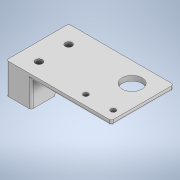
# Autodesk Inventor part: SwerveDriveBracket_B
Saved by Autodesk Inventor 2022.3 (Build 263350000, 350)
## iProperties
Created: 2022-06-17
Part Number: SwerveDriveBracket_B
Material: Generic
Document SubType Name: Modeling
Designer: Robert Nies
Density: 1 g/cm^3
Appearance: Default
Author: Robert Nies
Autodesk Inventor part; units mm, degrees
ref_plane "YZ Plane" through (0, 0, 0) normal (1, 0, 0) x (0, 1, 0)
ref_plane "XZ Plane" through (0, 0, 0) normal (0, 1, 0) x (-1, 0, 0)
ref_plane "XY Plane" through (0, 0, 0) normal (0, 0, 1) x (1, 0, 0)
sketch "Sketch1" plane through (0, 0, 0) normal (0, 1, 0) x (-1, 0, 0)
  line L0 (0, 0) -> (67.31, 0)
  line L1 (67.31, 0) -> (67.31, -40.005)
  line L2 (67.31, -40.005) -> (0, -40.005)
  line L3 (0, -40.005) -> (0, 0)
  dimension "d0" = 40.005
  dimension "d1" = 67.31
  constraints: 8 end point, 2 parallel, 1 horizontal, 1 perpendicular
  measures "d0" distance of L0.end L1.end
  measures "d1" distance of L1.end L2.end
extrude "Extrusion1" add sketch "Sketch1" along normal blind 3.175
sketch "Sketch2" plane through (0, 3.175, 0) normal (0, 1, 0) x (1, 0, 0)
  circle A0 centre (-13.97, 27.305) radius 6.35
  line L0 (0, 0) -> (0, 40.005) projected
  line L1 (-67.31, 0) -> (0, 0) projected
  line L2 (0, 40.005) -> (-67.31, 40.005) projected
  circle A1 centre (-5.08, 6.35) radius 1.5875
  circle A2 centre (-22.68, 6.35) radius 1.5875
  dimension "d4" = 13.97
  dimension "d28" = 12.7
  dimension "d29" = 12.7
  dimension "d30" = 3.175
  dimension "d31" = 3.175
  dimension "d32" = 5.08
  dimension "d33" = 17.6
  dimension "d34" = 6.35
  dimension "d35" = 6.35
  constraints: 3 centre point
  measures "d4" distance from line of L0 A0.centre
  measures "d28" distance from line of L2 A0.centre
  measures "d29" diameter of A0
  measures "d30" diameter of A1
  measures "d31" diameter of A2
  measures "d32" distance from line of L0 A1.centre
  measures "d33" distance of A1.centre A2.centre
  measures "d34" distance from line of L1 A1.centre
  measures "d35" distance from line of L1 A2.centre
extrude "Extrusion2" cut sketch "Sketch2" against normal blind 6.35
sketch "Sketch3" plane through (0, 0, 0) normal (0, -1, 0) x (1, 0, 0)
  line L0 (0, -40.005) -> (-67.31, -40.005) projected
  line L1 (-67.31, 0) -> (0, 0) projected
  line L2 (-67.31, -40.005) -> (-51.435, -40.005)
  line L3 (-51.435, -40.005) -> (-51.435, 0)
  line L4 (-51.435, 0) -> (-67.31, 0)
  line L5 (-67.31, 0) -> (-67.31, -40.005)
  point P0 (-67.31, 0)
  dimension "d8" = 15.875
  constraints: 8 end point, 2 parallel, 1 horizontal, 1 perpendicular, 1 point on line
  measures "d8" distance of L4.end L3.end
extrude "Extrusion3" add sketch "Sketch3" along normal blind 16.51
sketch "Sketch4" plane through (-67.31, 3.175, -40.005) normal (-1, 0, 0) x (0, 0, 1)
  line L0 (40.005, -19.685) -> (0, -19.685) projected
  circle A0 centre (20.0025, -19.685) radius 6.35
  point P0 (40.005, -3.175)
  point P1 (13.6525, -19.685)
  point P2 (26.3525, -19.685)
  dimension "d11" = 12.7
  constraints: 1 centre point, 1 midpoint
  measures "d11" diameter of A0
extrude "Extrusion4" cut sketch "Sketch4" against normal blind 6.35 contours L0 A0 picked at (22.0577, -19.1784)
sketch "Sketch5" plane through (-60.96, 3.175, -40.005) normal (-1, 0, 0) x (0, 0, 1)
  line L0 (26.3525, -19.685) -> (13.6525, -19.685) projected
  line L1 (20.0025, -19.685) -> (20.0025, -3.683)
  circle A0 centre (20.0025, -3.683) radius 3.175
  arc A1 (26.3525, -19.685) -> (13.6525, -19.685) centre (20.0025, -19.685) ccw projected
  line L2 (24.765, -15.4849) -> (15.24, -15.4849)
  line L3 (24.765, -15.4849) -> (23.1501, -3.267)
  line L4 (15.24, -15.4849) -> (16.8549, -3.267)
  point P0 (40.005, -3.175)
  dimension "d14" = 16.002
  dimension "d15" = 6.35
  dimension "d16" = 9.525
  constraints: 8 end point, 4 point on circle, 2 tangent, 1 centre point, 1 coincident, 1 horizontal, 1 midpoint, 1 vertical
  measures "d14" distance of L1.start L1.end
  measures "d15" diameter of A0
  measures "d16" distance of L2.start L2.end
extrude "Extrusion5" cut sketch "Sketch5" along normal blind 2.54 contours A1 L1 A0 L3 | A1 L4 A0 L1 | A0
sketch "Sketch6" plane through (0, 3.175, 0) normal (0, 1, 0) x (1, 0, 0)
  circle A0 centre (-55.88, 28.575) radius 2.1828
  circle A1 centre (-55.88, 9.525) radius 2.1828
  line L0 (-67.31, 40.005) -> (-67.31, 0) projected
  line L1 (-67.31, 0) -> (0, 0) projected
  dimension "d19" = 4.3656
  dimension "d20" = 4.3656
  dimension "d21" = 11.43
  dimension "d22" = 11.43
  dimension "d23" = 19.05
  dimension "d24" = 9.525
  constraints: 2 centre point
  measures "d19" diameter of A0
  measures "d20" diameter of A1
  measures "d21" distance from line of L0 A1.centre
  measures "d22" distance from line of L0 A0.centre
  measures "d23" distance of A1.centre A0.centre
  measures "d24" distance from line of L1 A1.centre
extrude "Extrusion6" cut sketch "Sketch6" against normal blind 25.4
fillet "Fillet1" radius 1.27 9 edges at (0, 0, -20.0025) (-25.7175, 0, 0) (-25.7175, 0, -40.005) (-51.435, -8.255, 0) (0, 1.5875, 0) (0, 1.5875, -40.005) (-67.31, -6.6675, -40.005) (-51.435, -8.255, -40.005) (-67.31, -6.6675, 0)
sketch "Sketch7" plane through (-67.31, -16.51, -20.0025) normal (-1, 0, 0) x (0, 0, 1)
  line L0 (-18.7325, 0) -> (18.7325, 0) projected
  circle A0 centre (0, 0) radius 4.7625
  point P0 (20.0025, 16.51)
  point P1 (4.7625, 0)
  point P2 (-4.7625, 0)
  dimension "d38" = 9.525
  constraints: 1 centre point, 1 midpoint
  measures "d38" diameter of A0
extrude "Extrusion7" cut sketch "Sketch7" against normal blind 25.4 contours A0 L0 picked at (1.1883, 1.0527)
body "Solid1"
